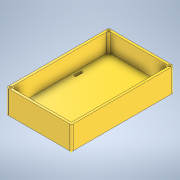
# Autodesk Inventor part: SUPERIOR MODEL2
Saved by Autodesk Inventor 2020 (Build 240168000, 168)
## iProperties
Created: 2022-05-31
Part Number: SUPERIOR MODEL2
Material: Generic
Document SubType Name: Modeling
Designer: juanc
Density: 1 g/cm^3
Appearance: Default
Author: juanc
Autodesk Inventor part; units mm, degrees
ref_plane "YZ Plane" through (0, 0, 0) normal (1, 0, 0) x (0, 1, 0)
ref_plane "XZ Plane" through (0, 0, 0) normal (0, 1, 0) x (-1, 0, 0)
ref_plane "XY Plane" through (0, 0, 0) normal (0, 0, 1) x (1, 0, 0)
sketch "Sketch1" plane through (0, 0, 0) normal (0, 1, 0) x (-1, 0, 0)
  line L0 (0, 0) -> (70, 0)
  line L1 (70, 0) -> (70, -110)
  line L2 (70, -110) -> (0, -110)
  line L3 (0, -110) -> (0, 0)
  line L4 (2.5, -2.49) -> (67.5, -2.49)
  line L5 (67.5, -2.49) -> (67.5, -107.49)
  line L6 (67.5, -107.49) -> (2.5, -107.49)
  line L7 (2.5, -107.49) -> (2.5, -2.49)
  line L8 (67.5, -54.99) -> (2.5, -54.99) construction
  line L9 (67.5, -54.99) -> (63.6, -54.99) construction
  line L10 (63.6, -54.99) -> (63.6, -71.2) construction
  line L11 (63.6, -71.2) -> (67.5, -71.2) construction
  line L12 (67.5, -71.2) -> (67.5, -54.99) construction
  line L13 (63.6, -68.2) -> (63.6, -74.2) construction
  line L14 (62.35, -68.2) -> (62.35, -74.2)
  line L15 (64.85, -74.2) -> (64.85, -68.2)
  arc A0 (64.85, -68.2) -> (62.35, -68.2) centre (63.6, -68.2) ccw
  arc A1 (62.35, -74.2) -> (64.85, -74.2) centre (63.6, -74.2) ccw
  line L16 (63.6, -71.2) -> (63.6, -87.6) construction
  line L17 (2.5, -87.6) -> (6.05, -87.6) construction
  line L18 (6.05, -84.6) -> (6.05, -90.6) construction
  line L19 (4.8, -84.6) -> (4.8, -90.6)
  line L20 (7.3, -90.6) -> (7.3, -84.6)
  arc A2 (7.3, -84.6) -> (4.8, -84.6) centre (6.05, -84.6) ccw
  arc A3 (4.8, -90.6) -> (7.3, -90.6) centre (6.05, -90.6) ccw
  line L21 (67.5, -2.49) -> (63.6, -2.49) construction
  line L22 (63.6, -2.49) -> (63.6, -18.7) construction
  line L23 (63.6, -18.7) -> (67.5, -18.7) construction
  line L24 (67.5, -18.7) -> (67.5, -2.49) construction
  line L25 (63.6, -18.7) -> (63.6, -35.1) construction
  line L26 (2.5, -35.1) -> (6.05, -35.1) construction
  line L27 (63.6, -15.7) -> (63.6, -21.7) construction
  line L28 (62.35, -15.7) -> (62.35, -21.7)
  line L29 (64.85, -21.7) -> (64.85, -15.7)
  arc A4 (64.85, -15.7) -> (62.35, -15.7) centre (63.6, -15.7) ccw
  arc A5 (62.35, -21.7) -> (64.85, -21.7) centre (63.6, -21.7) ccw
  line L30 (6.05, -32.1) -> (6.05, -38.1) construction
  line L31 (4.8, -32.1) -> (4.8, -38.1)
  line L32 (7.3, -38.1) -> (7.3, -32.1)
  arc A6 (7.3, -32.1) -> (4.8, -32.1) centre (6.05, -32.1) ccw
  arc A7 (4.8, -38.1) -> (7.3, -38.1) centre (6.05, -38.1) ccw
  point P0 (35, -55)
  dimension "d0" = 70
  dimension "d1" = 110
  dimension "d2" = 65
  dimension "d3" = 105
  dimension "d4" = 52.5
  dimension "d5" = 52.5
  dimension "d6" = 3.9
  dimension "d7" = 16.21
  dimension "d8" = 3
  dimension "d9" = 2.5
  dimension "d10" = 16.4
  dimension "d11" = 3.55
  dimension "d12" = 3
  dimension "d13" = 2.5
  dimension "d14" = 19.89
  dimension "d15" = 16.4
  dimension "d16" = 3.9
  dimension "d17" = 16.21
  dimension "d18" = 16.4
  dimension "d19" = 3.55
  dimension "d20" = 3
  dimension "d21" = 2.5
  dimension "d22" = 3
  dimension "d23" = 2.5
  constraints: 74 end point, 16 point on circle, 16 tangent, 12 parallel, 8 centre point, 6 midpoint, 6 perpendicular, 4 horizontal, 3 point on line, 3 vertical
  measures "d0" distance of L1.end L2.end
  measures "d1" distance of L0.end L1.end
  measures "d2" distance of L5.end L6.end
  measures "d3" distance of L4.end L5.end
  measures "d4" distance between parallel lines of L6 L8
  measures "d5" distance between parallel lines of L4 L8
  measures "d6" distance of L11.end L10.end
  measures "d7" distance of L10.end L9.end
  measures "d8" distance of L10.end L13.end
  measures "d9" diameter of A1
  measures "d10" distance of L10.end L16.end
  measures "d11" distance of L17.start L17.end
  measures "d12" distance of L17.end L18.end
  measures "d13" diameter of A3
  measures "d14" distance from line of L6 L17.end
  measures "d15" vertical distance of L17.end L10.end
  measures "d16" distance of L23.end L22.end
  measures "d17" distance of L22.end L21.end
  measures "d18" distance of L22.end L25.end
  measures "d19" distance of L26.start L26.end
  measures "d20" distance of L22.end L27.end
  measures "d21" diameter of A5
  measures "d22" distance of L26.end L30.end
  measures "d23" diameter of A7
extrude "Extrusion1" add sketch "Sketch1" along normal blind 25 contours L0 L1 L2 L3
extrude "Extrusion2" add sketch "Sketch1" along normal blind 5 contours L4 L5 L6 L7
sketch "Sketch2" plane through (0, 0, 0) normal (0, -1, 0) x (1, 0, 0)
  line L0 (-63.6, -21.7) -> (-63.6, -15.7) construction
  line L1 (-61.6, -21.7) -> (-61.6, -15.7)
  line L2 (-65.6, -15.7) -> (-65.6, -21.7)
  arc A0 (-65.6, -21.7) -> (-61.6, -21.7) centre (-63.6, -21.7) ccw
  arc A1 (-61.6, -15.7) -> (-65.6, -15.7) centre (-63.6, -15.7) ccw
  line L3 (-6.0099, -38.1033) -> (-6.0099, -32.1033) construction
  line L4 (-4.0099, -38.1033) -> (-4.0099, -32.1033)
  line L5 (-8.0099, -32.1033) -> (-8.0099, -38.1033)
  arc A2 (-8.0099, -38.1033) -> (-4.0099, -38.1033) centre (-6.0099, -38.1033) ccw
  arc A3 (-4.0099, -32.1033) -> (-8.0099, -32.1033) centre (-6.0099, -32.1033) ccw
  line L6 (-63.6, -74.2793) -> (-63.6, -68.2793) construction
  line L7 (-61.6, -74.2793) -> (-61.6, -68.2793)
  line L8 (-65.6, -68.2793) -> (-65.6, -74.2793)
  arc A4 (-65.6, -74.2793) -> (-61.6, -74.2793) centre (-63.6, -74.2793) ccw
  arc A5 (-61.6, -68.2793) -> (-65.6, -68.2793) centre (-63.6, -68.2793) ccw
  line L9 (-6.0099, -90.6) -> (-6.0099, -84.6) construction
  line L10 (-4.8, -90.6) -> (-4.8, -84.6) projected
  line L11 (-4.0099, -90.6) -> (-4.0099, -84.6)
  line L12 (-8.0099, -84.6) -> (-8.0099, -90.6)
  arc A6 (-8.0099, -90.6) -> (-4.0099, -90.6) centre (-6.0099, -90.6) ccw
  arc A7 (-4.0099, -84.6) -> (-8.0099, -84.6) centre (-6.0099, -84.6) ccw
  line L13 (-6.0099, -87.6) -> (-0.0099, -87.6) construction
  point P0 (0, 0)
  point P1 (-63.6, -18.7)
  point P2 (-6.0099, -35.1033)
  point P3 (-63.6, -71.2793)
  dimension "d28" = 3
  dimension "d29" = 4
  dimension "d30" = 3
  dimension "d31" = 4
  dimension "d32" = 3
  dimension "d33" = 4
  dimension "d34" = 3
  dimension "d35" = 90
  dimension "d36" = 4
  constraints: 34 end point, 16 point on circle, 16 tangent, 8 centre point, 5 parallel, 4 midpoint, 3 vertical, 1 horizontal, 1 perpendicular
  measures "d28" distance of point (-63.6, -18.7) L0.end
  measures "d29" diameter of A1
  measures "d30" distance of point (-6.01, -35.103) L3.end
  measures "d31" diameter of A3
  measures "d32" distance of point (-63.6, -71.279) L6.end
  measures "d33" diameter of A5
  measures "d34" distance of L13.start L9.end
  measures "d35" angle of L13 L9
  measures "d36" diameter of A7
extrude "Extrusion3" cut sketch "Sketch2" against normal blind 1
sketch "Sketch3" plane through (0, 25, 0) normal (0, 1, 0) x (1, 0, 0)
  line L0 (-67.5, 2.49) -> (-67.5, 107.49) projected
  circle A0 centre (-67.5, 2.49) radius 2.5
  line L1 (-70, 2) -> (-70, 108) projected
  circle A1 centre (-67.5, 107.477) radius 2.5
  line L2 (-67.5, 107.49) -> (-2.5, 107.49) projected
  circle A2 centre (-2.5, 107.49) radius 2.5
  point P0 (0, 0)
  dimension "d40" = 5
  constraints: 3 centre point, 1 tangent
  measures "d40" diameter of A2
extrude "Extrusion4" add sketch "Sketch3" against normal blind 24 contours A0 | A1 L2 L0 | L0 L2 A1 | A2
sketch "Sketch5" plane through (0, 0, 0) normal (0, -1, 0) x (1, 0, 0)
  arc A0 (-2.5, -104.99) -> (-5, -107.49) centre (-2.5, -107.49) ccw projected
  arc A1 (-65, -107.49) -> (-67.5, -104.977) centre (-67.5, -107.477) ccw projected
  arc A2 (-67.5, -4.99) -> (-65, -2.49) centre (-67.5, -2.49) ccw projected
  point P0 (0, 0)
  constraints: 3 coincident
hole "Hole1" at (-2.5, 0, -107.49) at (-67.5, 0, -107.477) at (-67.5, 0, -2.49) direction (0, 1, 0) diameter 3 depth 40 tip angle 118 counterbore diameter 3.5 counterbore depth 2
fillet "Fillet2" radius 2 4 edges at (-70, 12.5, 0) (-70, 12.5, -110) (0, 12.5, -110) (0, 12.5, 0)
sketch "Sketch6" plane through (0, 0, 0) normal (0, -1, 0) x (1, 0, 0)
  line L0 (-19.0093, -31.0437) -> (-19.0093, -43.6077) construction
  line L1 (-19.0093, -43.6077) -> (-93.3266, -43.6077) construction
  line L2 (-93.3266, -43.6077) -> (-93.3266, -31.0437) construction
  line L3 (-93.3266, -31.0437) -> (-19.0093, -31.0437) construction
  line L4 (-32.1283, -26.5619) -> (-32.1283, -53.8239) construction
  line L5 (-32.1283, -53.8239) -> (-124.1375, -53.8239) construction
  line L6 (-124.1375, -53.8239) -> (-124.1375, -26.5619) construction
  line L7 (-124.1375, -26.5619) -> (-32.1283, -26.5619) construction
  line L8 (-45.7196, -50.7865) -> (-45.7196, -85.058) construction
  line L9 (-45.7196, -85.058) -> (-48.896, -85.058) construction
  line L10 (-48.896, -85.058) -> (-48.896, -50.7865) construction
  line L11 (-48.896, -50.7865) -> (-45.7196, -50.7865) construction
  point P0 (0, 0)
  constraints: 6 other
body "Solid1"
